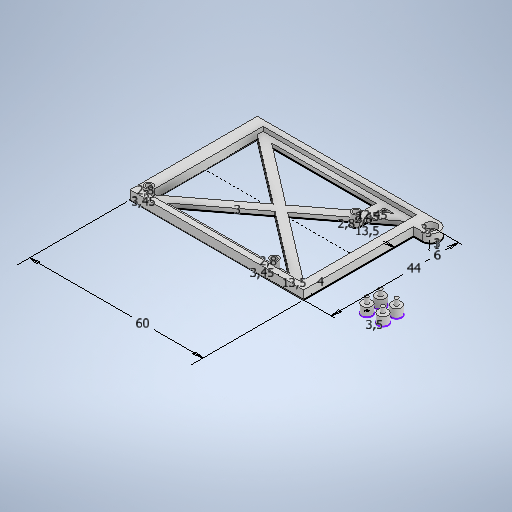
# Autodesk Inventor part: HållareV.2
Saved by Autodesk Inventor 2025.2 (Build 292293000, 293)
## iProperties
Created: 2025-01-21
Part Number: HållareV.2
Material: Generic
Document SubType Name: Modeling
Designer: 24oscnor
Density: 1 g/cm^3
Appearance: Default
Author: 24oscnor
Autodesk Inventor part; units mm, degrees
ref_plane "YZ Plane" through (0, 0, 0) normal (1, 0, 0) x (0, 1, 0)
ref_plane "XZ Plane" through (0, 0, 0) normal (0, 1, 0) x (-1, 0, 0)
ref_plane "XY Plane" through (0, 0, 0) normal (0, 0, 1) x (1, 0, 0)
sketch "Sketch1" plane through (0, 0, 0) normal (0, 1, 0) x (-1, 0, 0)
  line L0 (0, 0) -> (60, 0)
  line L1 (60, 0) -> (60, 44)
  line L2 (60, 44) -> (0, 44)
  line L3 (0, 44) -> (0, 0)
  line L4 (4, 4) -> (56, 4)
  line L5 (56, 4) -> (56, 40)
  line L6 (56, 40) -> (4, 40)
  line L7 (4, 40) -> (4, 4)
  line L8 (56, 40) -> (8.9377, 4)
  line L9 (4, 4) -> (51.0623, 40)
  line L10 (56, 22) -> (4, 22) construction
  line L11 (56, 4) -> (8.9377, 40)
  line L12 (4, 40) -> (51.0623, 4)
  circle A0 centre (13.5, 12.45) radius 1.4
  line L13 (14.9, 12.45) -> (12.1, 12.45)
  line L14 (12.1, 12.45) -> (12.1, 4)
  line L15 (12.1, 4) -> (14.9, 4)
  line L16 (14.9, 4) -> (14.9, 12.45)
  circle A1 centre (57, 40.55) radius 1.4
  circle A2 centre (13.5, 40.55) radius 1.4002
  circle A3 centre (-14.9003, 37.017) radius 1.75
  circle A4 centre (-14.9003, 32.3222) radius 1.75
  circle A5 centre (-20.4624, 32.3222) radius 1.75
  circle A6 centre (-20.4624, 37.017) radius 1.75
  circle A7 centre (-3, 3) radius 3
  line L17 (0, 0) -> (-3, 0)
  line L18 (-3, 6) -> (0, 6)
  circle A8 centre (-3, 3) radius 2
  circle A9 centre (-3, 3) radius 1.5
  point P0 (32.4689, 22)
  point P1 (55.7926, 39.8414)
  point P2 (56, 39.5702)
  point P3 (30, 23.8885)
  point P4 (8.9377, 40)
  point P5 (12.2124, 40)
  point P6 (14.7876, 40)
  point P7 (30, 20.1115)
  point P8 (27.5311, 22)
  point P9 (14.8952, 12.3342)
  point P10 (12.1, 10.196)
  point P11 (14.9, 8.5608)
  point P12 (12.1, 6.419)
  point P13 (0, 3)
  dimension "d6" = 2.8
  dimension "d0" = 60
  dimension "d1" = 44
  dimension "d3" = 3
  dimension "d4" = 4
  dimension "d7" = 13.5
  dimension "d8" = 12.45
  dimension "d9" = 2.8
  dimension "d10" = 8.45
  dimension "d11" = 3.45
  dimension "d12" = 3
  dimension "d13" = 2.8
  dimension "d14" = 3.45
  dimension "d15" = 13.5
  dimension "d16" = 2.8004
  dimension "d37" = 3.5
  dimension "d56" = 6
  dimension "d57" = 3
  dimension "d58" = 3
  dimension "d59" = 1
  dimension "d60" = 3
  constraints: 38 end point, 9 centre point, 7 parallel, 4 perpendicular, 4 point on line, 2 coincident, 2 horizontal, 2 midpoint, 2 point on circle, 2 symmetric about line, 2 tangent, 6 other
  measures "d0" distance of L1.end L2.end
  measures "d1" distance between parallel lines of L0 L2
  measures "d3" distance between parallel lines of L8 L9
  measures "d4" distance between parallel lines of L7 L3
  measures "d7" distance from line of point (13.5, 12.45) L3
  measures "d8" distance from line of L0 point (13.5, 12.45)
  measures "d9" distance between parallel lines of L16 L14
  measures "d10" distance between parallel lines of L4 L13
  measures "d11" distance from line of L2 A1.centre
  measures "d12" distance from line of L1 A1.centre
  measures "d13" diameter of A1
  measures "d14" distance from line of L2 A2.centre
  measures "d15" distance from line of L3 A2.centre
  measures "d16" diameter of A2
  measures "d37" diameter of A3
  measures "d56" diameter of A7
  measures "d57" distance from line of L3 A7.centre
  measures "d58" distance from line of L0 A7.centre
  measures "d59" radial gap between concentric circles of A7 A8
  measures "d60" diameter of A9
extrude "Extrusion1" add sketch "Sketch1" along normal blind 3 contours L3 L2 L1 L0 | L17 A7 L3 | A7 L18 L3 | A7 | L9 L14 L8 L4 | L6 L11 L9 L12 | L14 A0 L9 | L9 A0 L16 L8 L14 | L14 L8 L16 L4 | L12 L8 L16 L9 | L9 L11 L8 L12 | L9 L6 A1 L8 L11 | L8 L11 L4 L12
extrude "Extrusion2" add sketch "Sketch1" along normal blind 4 contours A0 L13 L9 | L9 A0 | A0 L13 | A2 L6 | L6 A2 | A1 L5 L6 | L6 L8 A1 | L8 L5 A1
sketch "Sketch2" plane through (0, 3, 0) normal (0, 1, 0) x (1, 0, 0)
  line L0 (-4, -40) -> (-27.5311, -22) projected
  line L1 (-4, -40) -> (-56, -40)
  line L2 (-56, -40) -> (-56, -42)
  line L3 (-56, -42) -> (-4, -42)
  line L4 (-4, -42) -> (-4, -40)
  line L5 (-51.0623, -4) -> (-56, -4)
  line L6 (-32.4689, -22) -> (-55.7926, -39.8414) projected
  line L7 (-32.4689, -22) -> (-55.7926, -39.8414)
  line L8 (-56, -40) -> (-32.4689, -22)
  line L9 (-32.4689, -22) -> (-56, -40)
  line L10 (-51.0623, -40) -> (-30, -23.8885) projected
  line L11 (-27.5311, -22) -> (-4, -40)
  line L12 (-14.9, -8.5608) -> (-30, -20.1115) projected
  line L13 (-30, -20.1115) -> (-14.9, -8.5608)
  line L14 (-14.9, -8.5608) -> (-30, -20.1115)
  line L15 (-14.9, -4) -> (-14.9, -8.5608) projected
  line L16 (-4, -4) -> (-4, -40) projected
  circle A0 centre (-13.5, -12.45) radius 1.4 projected
  circle A1 centre (-13.5, -12.45) radius 1.4
  line L17 (-14.9, -3) -> (-4, -3)
  line L18 (-14.9, -3) -> (-56, -3)
  line L19 (-56, -3) -> (-56, -4)
  line L20 (-3, -42) -> (-3, -3)
  line L21 (-3, -3) -> (-4, -3)
  line L22 (-3, -42) -> (-4, -42)
  line L23 (-4, -40) -> (-27.5311, -22)
  line L24 (-12.1, -12.45) -> (-12.1, -10.196) projected
  line L25 (-12.1, -10.196) -> (-4, -4)
  line L26 (-4, -40) -> (-4, -4)
  line L27 (-4, -40) -> (-27.5311, -22)
  line L28 (-30, -20.1115) -> (-51.0623, -4)
  line L29 (-56, -4) -> (-32.4689, -22)
  line L30 (-32.4689, -22) -> (-56, -40)
  line L31 (-30, -23.8885) -> (-51.0623, -40)
  line L32 (-30, -23.8885) -> (-8.9377, -40)
  line L33 (-27.5311, -22) -> (-14.8952, -12.3342) projected
  line L34 (-27.5311, -22) -> (-14.8952, -12.3342)
  line L35 (-27.5311, -22) -> (-14.8952, -12.3342)
  line L36 (-12.1, -10.196) -> (-12.1, -12.45)
  line L37 (-51.0623, -4) -> (-14.9, -4)
  arc A2 (-14.7876, -40) -> (-12.2124, -40) centre (-13.5, -40.55) ccw projected
  circle A3 centre (-13.5, -40.55) radius 1.4002
  arc A4 (-56, -39.5702) -> (-55.7926, -39.8414) centre (-57, -40.55) ccw projected
  circle A5 centre (-57, -40.55) radius 1.4
  line L38 (-3, -3) -> (-3, -2)
  line L39 (-3, -2) -> (-56, -2)
  line L40 (-56, -2) -> (-56, -3)
  point P0 (0, 0)
  point P1 (-4, -41)
  point P2 (-56, -41.5298)
  dimension "d23" = 2
  dimension "d25" = 9.45
  dimension "d26" = 1
  dimension "d65" = 1
  constraints: 66 end point, 9 collinear, 7 parallel, 6 horizontal, 4 perpendicular, 3 coincident, 3 point on line, 2 centre point, 2 vertical, 1 horizontal alignment, 1 midpoint, 2 other
  measures "d23" distance between parallel lines of L3 L1
  measures "d25" distance from line of A0.centre L17
  measures "d26" distance from line of point (-4, -41) L20
  measures "d65" distance between parallel lines of L18 L39
extrude "Extrusion4" cut sketch "Sketch2" against normal blind 1.5 contours L4 L3 L2 A4 L1 A2 | L1 L32 L10 A4 L6 L29 L19 L18 L17 L21 L20 L22 L4 | L21 L17 L18 L40 L39 L38
sketch "Sketch3" plane through (-13.5, 4, 40.55) normal (0, 1, 0) x (1, 0, 0)
  circle A0 centre (0, 0) radius 0.9
  circle A1 centre (0, 0) radius 1.4002 projected
  circle A2 centre (-43.5, 0) radius 0.9
  circle A3 centre (-43.5, 0) radius 1.4 projected
  circle A4 centre (0, 28.1) radius 0.9
  circle A5 centre (0, 28.1) radius 1.4 projected
  point P0 (13.5, 40.55)
  dimension "d29" = 1.8
  dimension "d30" = 0.5002
  dimension "d31" = 1.8
  dimension "d32" = 0
  dimension "d33" = 1.8
  dimension "d34" = 0
  constraints: 3 centre point
  measures "d29" diameter of A0
  measures "d30" radial gap between concentric circles of A1 A0
  measures "d31" diameter of A2
  measures "d32" distance of A3.centre A2.centre
  measures "d33" diameter of A4
  measures "d34" distance of A5.centre A4.centre
extrude "Extrusion5" cut sketch "Sketch3" against normal through all contours A0 | A2 | A4
extrude "Extrusion6" add sketch "Sketch1" along normal blind 3 contours A3 | A4 | A5 | A6
sketch "Sketch4" plane through (25.079, 3, 37.017) normal (0, 1, 0) x (1, 0, 0)
  circle A0 centre (-10.1787, 4.6948) radius 0.65
  circle A1 centre (-10.1787, 4.6948) radius 1.75 projected
  circle A2 centre (-4.6166, 4.6948) radius 0.65
  circle A3 centre (-4.6166, 4.6948) radius 1.75 projected
  circle A4 centre (-10.1787, 0) radius 0.65
  circle A5 centre (-4.6166, 0) radius 0.65
  circle A6 centre (-10.1787, 0) radius 1.75 projected
  circle A7 centre (-4.6166, 0) radius 1.75 projected
  point P0 (-25.079, 37.017)
  point P1 (0, 0)
  dimension "d40" = 0
  dimension "d41" = 1.3
  dimension "d42" = 0
  dimension "d43" = 1.3
  dimension "d44" = 0
  dimension "d45" = 0
  dimension "d50" = 0
  dimension "d53" = 1.3
  dimension "d54" = 1.3
  constraints: 4 centre point
  measures "d40" distance of A1.centre A0.centre
  measures "d41" diameter of A0
  measures "d42" distance of A3.centre A2.centre
  measures "d43" diameter of A2
  measures "d44" distance of A6.centre A4.centre
  measures "d45" distance of A7.centre A5.centre
  measures "d50" distance of A1.centre A0.centre
  measures "d53" diameter of A4
  measures "d54" diameter of A5
extrude "Extrusion7" add sketch "Sketch4" along normal blind 2 contours A0 | A2 | A4 | A5
extrude "Extrusion8" add sketch "Sketch1" along normal blind 1 contours A8
equation "\"d31\" = d29"
equation "\"d33\" = d29"
body "Solid1"
